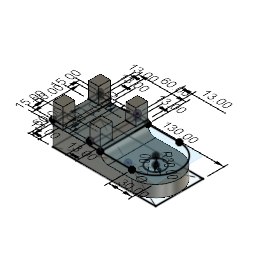
fus3603 (Autodesk Fusion 360 design; units mm, degrees)
Autodesk Fusion 360 part; units mm, degrees
sketch "Sketch1" plane through (0, 0, 0) normal (0, 0, 1) x (1, 0, 0) in component "Component"
  line L0 (65, -30) -> (-65, -30)
  line L1 (-65, -30) -> (-65, 30)
  line L2 (-65, 30) -> (65, 30)
  line L3 (65, 30) -> (65, -30)
  line L4 (65, -30) -> (-65, 30) construction
  line L5 (-65, -30) -> (65, 30) construction
  dimension "d1" = 130
  dimension "d2" = 60
  constraint horizontal L0
  constraint perpendicular L0 L1
  constraint parallel L0 L2
  constraint parallel L1 L3
  constraint coincident L4 origin
  constraint coincident L5 origin
  measures "d1" distance of L1.end L2.end
  measures "d2" distance of L0.end L1.end
extrude "Extrude1" add sketch "Sketch1" along normal blind 25 in component "Component"
sketch "Sketch2" plane through (0, 0, 25) normal (0, 0, 1) x (-1, 0, 0) in component "Component"
  line L0 (-65, -30) -> (65, -30)
  line L1 (65, -30) -> (65, 30)
  line L2 (65, 30) -> (-65, 30)
  line L3 (-65, 30) -> (-65, -30)
  line L4 (65, -30) -> (52, -30)
  line L5 (52, -30) -> (52, 30)
  line L6 (52, 30) -> (65, 30)
  line L7 (65, 30) -> (65, -30)
  line L8 (18, -30) -> (5, -30)
  line L9 (5, -30) -> (5, 30)
  line L10 (5, 30) -> (18, 30)
  line L11 (18, 30) -> (18, -30)
  dimension "d5" = 13
  dimension "d6" = 60
  dimension "d7" = 13
  dimension "d8" = 60
  dimension "d9" = 60
  constraint horizontal L4
  constraint vertical L5
  constraint horizontal L6
  constraint vertical L7
  constraint coincident L0.end L1.start
  constraint horizontal L8
  constraint vertical L9
  constraint horizontal L10
  constraint vertical L11
  constraint coincident L0 L8.start
  measures "d5" distance of L0.end L4.end
  measures "d6" distance of L0.end L1.end
  measures "d7" distance of L8.start L8.end
  measures "d8" distance of L8.start L10.end
  measures "d9" distance of L0.end L8.end
extrude "Extrude2" add sketch "Sketch2" along normal blind 5 contours L0 L2 L8 L9 L10 L11 | L0 L1 L2 L4 L5 L6 L7 in component "Component"
sketch "Sketch3" plane through (0, 0, 30) normal (0, 0, 1) x (-1, 0, 0) in component "Component"
  line L0 (65, 30) -> (52, 30)
  line L1 (52, 30) -> (52, -30)
  line L2 (52, -30) -> (65, -30)
  line L3 (65, -30) -> (65, 30)
  line L4 (65, -30) -> (52, -30)
  line L5 (52, -30) -> (52, -15)
  line L6 (52, -15) -> (65, -15)
  line L7 (65, -15) -> (65, -30)
  line L8 (65, 30) -> (52, 30)
  line L9 (52, 30) -> (52, 15)
  line L10 (52, 15) -> (65, 15)
  line L11 (65, 15) -> (65, 30)
  line L12 (18, -30) -> (5, -30)
  line L13 (5, -30) -> (5, -15)
  line L14 (5, -15) -> (18, -15)
  line L15 (18, -15) -> (18, -30)
  line L16 (18, 30) -> (5, 30)
  line L17 (5, 30) -> (5, 15)
  line L18 (5, 15) -> (18, 15)
  line L19 (18, 15) -> (18, 30)
  point P0 (18, -30)
  point P1 (18, 30)
  dimension "d12" = 15
  dimension "d13" = 13
  dimension "d14" = 13
  dimension "d15" = 15
  dimension "d16" = 15
  dimension "d17" = 13
  dimension "d18" = 13
  dimension "d19" = 15
  constraint horizontal L4
  constraint vertical L5
  constraint horizontal L6
  constraint vertical L7
  constraint coincident L2.end L3.start
  constraint horizontal L8
  constraint vertical L9
  constraint horizontal L10
  constraint vertical L11
  constraint coincident L0.start L3.end
  constraint horizontal L12
  constraint vertical L13
  constraint horizontal L14
  constraint vertical L15
  constraint coincident P0 L12.start
  constraint horizontal L16
  constraint vertical L17
  constraint horizontal L18
  constraint vertical L19
  constraint coincident P1 L16.start
  measures "d12" distance of L2.end L6.end
  measures "d13" distance of L2.end L1.end
  measures "d14" distance of L0.start L0.end
  measures "d15" distance of L0.start L10.end
  measures "d16" distance of P0 L14.end
  measures "d17" distance of P0 L12.end
  measures "d18" distance of P1 L16.end
  measures "d19" distance of P1 L18.end
extrude "Extrude3" add sketch "Sketch3" along normal blind 20 contours L0 L1 L3 L8 L9 L10 L11 | L1 L2 L3 L4 L5 L6 L7 | L12 L13 L14 L15 | L16 L17 L18 L19 in component "Component"
sketch "Sketch4" plane through (0, 0, 25) normal (0, 0, 1) x (-1, 0, 0) in component "Component"
  line L0 (5, -30) -> (5, 30)
  line L1 (5, 30) -> (-65, 30)
  line L2 (-65, 30) -> (-65, -30)
  line L3 (-65, -30) -> (5, -30)
  arc A0 (-35, 30) -> (-35, -30) centre (-35, 0) ccw
  line L4 (5, -30) -> (-35, -30)
  line L5 (5, -30) -> (5, 30)
  line L6 (5, 30) -> (-35, 30)
  dimension "d22" = 30
  dimension "d23" = 30
  constraint tangent L2 A0
  constraint coincident L1 A0.start
  constraint coincident L3 A0.end
  constraint coincident L0.start L3.end
  constraint tangent A0 L4
  constraint coincident L0.end L1.start
  measures "d22" distance of L1.end A0.start
  measures "d23" radius of A0
extrude "Extrude4" cut sketch "Sketch4" against normal blind 10 contours L0 L1 L3 A0 L4 L5 L6 in component "Component"
extrude "Extrude5" cut 2 faces at (59.1061, -24.1061, 25) (59.1061, 24.1061, 25) along direction (0, 0, -1) blind 30 in component "Component"
sketch "Sketch5" plane through (0, 0, 15) normal (0, 0, 1) x (-1, 0, 0) in component "Component"
  line L0 (5, -30) -> (5, 30)
  line L1 (5, 30) -> (-35, 30)
  arc A0 (-35, 30) -> (-35, -30) centre (-35, 0) ccw
  line L2 (-35, -30) -> (5, -30)
  circle A1 centre (-35, 0) radius 11
  dimension "d28" = 22
  constraint concentric A0 A1
extrude "Extrude6" cut sketch "Sketch5" against normal up to surface (15 mm away) contours A1 in component "Component"
fillet "Fillet1" radius 10 1 edges at (-5, 0, 15) in component "Component"
sketch "Sketch6" plane through (-5, 0, 0) normal (1, 0, 0) x (0, 1, 0) in component "Component"
  line L0 (-30, 25) -> (30, 25)
  line L1 (30, 25) -> (30, 50)
  line L2 (30, 50) -> (15, 50)
  line L3 (15, 50) -> (15, 30)
  line L4 (15, 30) -> (-15, 30)
  line L5 (-15, 30) -> (-15, 50)
  line L6 (-15, 50) -> (-30, 50)
  line L7 (-30, 50) -> (-30, 25)
component "Component" placed x (1, 0, 0) y (0, 1, 0) z (0, 0, 1) at (0, 0, 0)
component "Component'" placed x (1, 0, 0) y (0, 1, 0) z (0, 0, 1) at (0, 0, 0)
